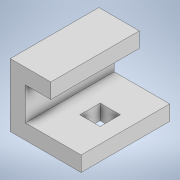
# Autodesk Inventor part: 2.1
Saved by Autodesk Inventor 2022 (Build 260153000, 153)
## iProperties
Created: 2023-04-17
Part Number: 2.1
Material: Genérico
Document SubType Name: Modeling
Designer: jpjoa
Density: 1 g/cm^3
Appearance: Padrão
Author: jpjoa
Autodesk Inventor part; units mm, degrees
ref_plane "YZ Plane" through (0, 0, 0) normal (1, 0, 0) x (0, 1, 0)
ref_plane "XZ Plane" through (0, 0, 0) normal (0, 1, 0) x (-1, 0, 0)
ref_plane "XY Plane" through (0, 0, 0) normal (0, 0, 1) x (1, 0, 0)
sketch "Esboço1" plane through (0, 0, 0) normal (0, 0, 1) x (1, 0, 0)
  line L0 (0, 0) -> (56, 0)
  line L1 (0, 0) -> (0, 50)
  line L2 (0, 50) -> (32, 50)
  line L3 (32, 38) -> (12, 38)
  line L4 (12, 38) -> (12, 12)
  line L5 (12, 12) -> (56, 12)
  line L6 (32, 50) -> (32, 38)
  line L7 (56, 12) -> (56, 0)
  dimension "d3" = 56
  dimension "d4" = 50
  dimension "d5" = 32
  dimension "d6" = 12
  constraints: 16 end point, 2 perpendicular, 2 vertical, 1 horizontal, 1 parallel, 2 other
  measures "d3" distance of L0.start L0.end
  measures "d4" distance of L0.start L1.end
  measures "d5" distance of L1.end L2.end
  measures "d6" distance between parallel lines of L1 L4
extrude "Extrusão1" add sketch "Esboço1" along normal blind 70
sketch "Esboço2" plane through (12, 12, 0) normal (0, 1, 0) x (1, 0, 0)
  line L0 (16, -43) -> (32, -43)
  line L1 (32, -43) -> (32, -27)
  line L2 (32, -27) -> (16, -27)
  line L3 (16, -27) -> (16, -43)
  line L4 (44, -70) -> (0, -70) projected
  line L5 (44, 0) -> (44, -70) projected
  point P0 (-12, 0)
  dimension "d9" = 16
  dimension "d10" = 16
  dimension "d11" = 27
  dimension "d13" = 12
  constraints: 8 end point, 2 parallel, 1 horizontal, 1 perpendicular
  measures "d9" distance of L2.end L1.end
  measures "d10" distance of L1.end L0.end
  measures "d11" distance between parallel lines of L4 L0
  measures "d13" distance between parallel lines of L5 L1
extrude "Extrusão2" cut sketch "Esboço2" against normal through all
